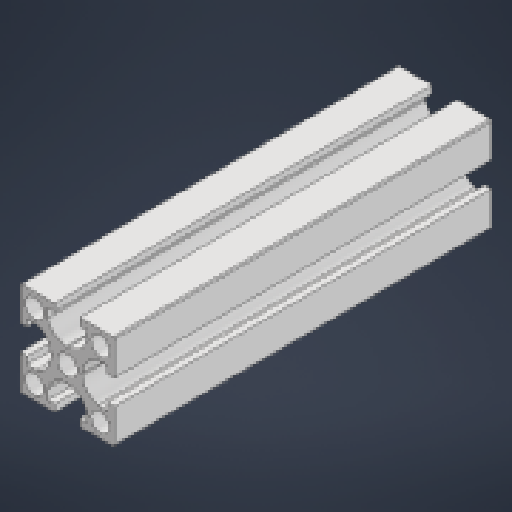
# Autodesk Inventor part: profile
Saved by Autodesk Inventor 2026.1 (Build 301233020, 233B)
## iProperties
Created: 2025-11-28
Part Number: profile
Material: 일반
Document SubType Name: Modeling
Designer: jaewook
Density: 1 g/cm^3
Appearance: 기본값
Author: jaewook
Autodesk Inventor part; units mm, degrees
ref_plane "YZ Plane" through (0, 0, 0) normal (1, 0, 0) x (0, 1, 0)
ref_plane "XZ Plane" through (0, 0, 0) normal (0, 1, 0) x (-1, 0, 0)
ref_plane "XY Plane" through (0, 0, 0) normal (0, 0, 1) x (1, 0, 0)
sketch "스케치1" plane through (0, 0, 0) normal (0, 0, 1) x (1, 0, 0)
  line L0 (9.7, -10) -> (-9.7, -10)
  line L1 (-10, -9.7) -> (-10, 9.7)
  line L2 (-9.7, 10) -> (9.7, 10)
  line L3 (10, 9.7) -> (10, -9.7)
  line L4 (10, -10) -> (-10, 10) construction
  line L5 (-10, -10) -> (10, 10) construction
  line L6 (7, -7) -> (-7, -7) construction
  line L7 (-7, -7) -> (-7, 7) construction
  line L8 (-7, 7) -> (7, 7) construction
  line L9 (7, 7) -> (7, -7) construction
  line L10 (7, -7) -> (-7, 7) construction
  line L11 (-7, -7) -> (7, 7) construction
  circle A0 centre (-7, 7) radius 2
  circle A1 centre (0, 0) radius 2.15
  arc A2 (9.7, -10) -> (10, -9.7) centre (9.7, -9.7) ccw
  arc A3 (-10, -9.7) -> (-9.7, -10) centre (-9.7, -9.7) ccw
  arc A4 (-9.7, 10) -> (-10, 9.7) centre (-9.7, 9.7) ccw
  arc A5 (10, 9.7) -> (9.7, 10) centre (9.7, 9.7) ccw
  line L12 (0, 10) -> (0, -10) construction
  line L13 (10, 0) -> (-10, 0) construction
  line L14 (2.65, -10) -> (-2.65, -10)
  line L15 (-2.65, -10) -> (-2.65, -8.5)
  line L16 (-2.65, -8.5) -> (2.65, -8.5)
  line L17 (2.65, -8.5) -> (2.65, -10)
  line L18 (4.15, -3.3) -> (-4.15, -3.3) construction
  line L19 (-4.15, -3.3) -> (-4.15, -8.5) construction
  line L20 (-4.15, -8.5) -> (4.15, -8.5)
  line L21 (4.15, -8.5) -> (4.15, -3.3) construction
  arc A6 (4.15, -6.4742) -> (-4.15, -6.4742) centre (0, -7.6) ccw
  line L22 (42.9153, -82.9009) -> (54.7664, -82.9009) construction
  line L23 (54.7664, -82.9009) -> (54.7664, -95.6544) construction
  line L24 (54.7664, -95.6544) -> (42.9153, -95.6544) construction
  line L25 (42.9153, -95.6544) -> (42.9153, -82.9009) construction
  arc A7 (44.9755, -91.1725) -> (50.2986, -91.1614) centre (47.6297, -87.6532) ccw
  line L26 (0, -3.1269) -> (-0.1768, -3.3036)
  line L27 (0, -3.1269) -> (0, -3.3) construction
  line L28 (0, -3.1269) -> (0.1731, -3.1269) construction
  line L29 (47.4573, -92.1078) -> (47.6389, -92.3063)
  line L30 (0, -3.1269) -> (0.1768, -3.3036)
  line L31 (-4.15, -6.4742) -> (-4.15, -8.5)
  line L32 (4.15, -8.5) -> (4.15, -6.4742)
  arc A8 (6.4742, 4.15) -> (6.4742, -4.15) centre (7.6, 0) ccw
  line L33 (8.5, 4.15) -> (6.4742, 4.15)
  line L34 (3.3, -4.15) -> (8.5, -4.15) construction
  line L35 (6.4742, -4.15) -> (8.5, -4.15)
  line L36 (8.5, -4.15) -> (8.5, 4.15)
  line L37 (10, -2.65) -> (8.5, -2.65)
  line L38 (8.5, 2.65) -> (10, 2.65)
  line L39 (3.1269, 0) -> (3.3036, -0.1768)
  line L40 (3.1269, 0) -> (3.3036, 0.1768)
  arc A9 (-4.15, 6.4742) -> (4.15, 6.4742) centre (0, 7.6) ccw
  line L41 (-4.15, 8.5) -> (-4.15, 6.4742)
  line L42 (4.15, 3.3) -> (4.15, 8.5) construction
  line L43 (4.15, 6.4742) -> (4.15, 8.5)
  line L44 (4.15, 8.5) -> (-4.15, 8.5)
  line L45 (2.65, 10) -> (2.65, 8.5)
  line L46 (-2.65, 8.5) -> (-2.65, 10)
  line L47 (0, 3.1269) -> (0.1768, 3.3036)
  line L48 (0, 3.1269) -> (-0.1768, 3.3036)
  arc A10 (-6.4742, -4.15) -> (-6.4742, 4.15) centre (-7.6, 0) ccw
  line L49 (-8.5, -4.15) -> (-6.4742, -4.15)
  line L50 (-3.3, 4.15) -> (-8.5, 4.15) construction
  line L51 (-6.4742, 4.15) -> (-8.5, 4.15)
  line L52 (-8.5, 4.15) -> (-8.5, -4.15)
  line L53 (-10, 2.65) -> (-8.5, 2.65)
  line L54 (-8.5, -2.65) -> (-10, -2.65)
  line L55 (-3.1269, 0) -> (-3.3036, 0.1768)
  line L56 (-3.1269, 0) -> (-3.3036, -0.1768)
  circle A11 centre (-7, -7) radius 2
  circle A12 centre (7, -7) radius 2
  circle A13 centre (7, 7) radius 2
  point P0 (3.3, 0)
  point P1 (0, 3.3)
  point P2 (-3.3, 0)
  point P3 (6.4742, -4.15)
  point P4 (4.15, 6.4742)
  point P5 (-6.4742, 4.15)
  point P6 (-4.15, -6.4742)
  dimension "d0" = 20
  dimension "d1" = 20
  dimension "d2" = 14
  dimension "d3" = 14
  dimension "d4" = 4
  dimension "d5" = 4.3
  dimension "d6" = 0.3
  dimension "d7" = 5.3
  dimension "d8" = 1.5
  dimension "d9" = 6.7
  dimension "d10" = 8.3
  dimension "d11" = 4.3
  dimension "d28" = 0.25
  dimension "d30" = 90
  dimension "d37" = 45
  dimension "d41" = 360
  dimension "d48" = 360
  constraints: 106 end point, 26 point on circle, 19 point on line, 14 centre point, 9 parallel, 9 tangent, 8 midpoint, 6 perpendicular, 5 horizontal, 3 equal radius, 2 coincident, 2 collinear, 1 horizontal alignment, 1 symmetric about line, 110 other
  measures "d0" distance of L4.end L5.end
  measures "d1" distance of L5.start L4.end
  measures "d2" distance of L7.end L8.end
  measures "d3" distance of L6.end L7.end
  measures "d4" diameter of A0
  measures "d5" diameter of A1
  measures "d6" radius of A2
  measures "d7" distance of L15.end L16.end
  measures "d8" distance of L14.end L15.end
  measures "d9" distance between parallel lines of L0 L18
  measures "d10" distance of L19.end L20.end
  measures "d11" radius of A6
  measures "d28" distance of L26.start L26.end
  measures "d30" angle of L27 L28
  measures "d37" angle of L12 L26
extrude "돌출1" add sketch "스케치1" along normal blind 80 contours L0 L17 L20 L32 A6 L30 L26 L31 L15 A3 L1 L54 L52 L49 A10 L56 L55 L51 L53 A4 L2 L46 L44 L41 A9 L48 L47 L43 L45 A5 L3 L38 L36 L33 A8 L40 L39 L35 L37 A2
